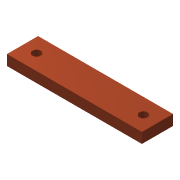
# Autodesk Inventor part: 17-0028-0035
Saved by Autodesk Inventor 2016 SP2 (Build 200236200, 236)
## iProperties
Category: IOP
Company: Universiteit van Amsterdam
Created: 2017-11-20
Part Number: 17-0028-0035
Material: Copper
Document SubType Name: Modeling
Designer: Daan Giesen
Density: 8.94 g/cm^3
Appearance: Copper - Satin
Project: Digital PID Loop
Cost Center: 17-0028
User Status: Work in Progress
Authority: Reichsöllner, Lukas
Description: Battery connector bar
Author: Daan Giesen
Title: Digital PID Loop
Revision Number: A
Autodesk Inventor part; units mm, degrees
ref_plane "YZ Plane" through (0, 0, 0) normal (1, 0, 0) x (0, 1, 0)
ref_plane "XZ Plane" through (0, 0, 0) normal (0, 1, 0) x (-1, 0, 0)
ref_plane "XY Plane" through (0, 0, 0) normal (0, 0, 1) x (1, 0, 0)
sketch "Sketch1" plane through (0, 0, 0) normal (0, 0, 1) x (1, 0, 0)
  line L0 (0, 21) -> (0, -21) construction
  line L1 (-91, 0) -> (91, 0) construction
  line L2 (65, -15) -> (-65, -15)
  line L3 (-65, -15) -> (-65, 15)
  line L4 (-65, 15) -> (65, 15)
  line L5 (65, 15) -> (65, -15)
  line L6 (65, -15) -> (-65, 15) construction
  line L7 (-65, -15) -> (65, 15) construction
  point P0 (0, 0)
  dimension "d4" = 130
  dimension "d5" = 30
  constraints: 12 end point, 2 midpoint, 2 parallel, 1 horizontal, 1 perpendicular
  measures "d4" distance of L3.end L4.end
  measures "d5" distance of L2.end L3.end
extrude "Extrusion3" add sketch "Sketch1" along normal mid plane 10
sketch "Sketch2" plane through (0, 0, -5) normal (0, 0, -1) x (-1, 0, 0)
  point P0 (0, 0)
  point P1 (-50.9, 0)
  point P2 (50.9, 0)
  dimension "d8" = 101.8
  dimension "d9" = 50.9
  constraints: 2 horizontal alignment
  measures "d8" distance of point (50.9, 0) point (-50.9, 0)
  measures "d9" distance of point (0, 0) point (-50.9, 0)
hole "Hole1" at (50.9, 0, -5) at (-50.9, 0, -5) direction (0, 0, 1) diameter 8.2 end through all
equation "\"d9\" = 0.5 * d8"
body "Solid3"
